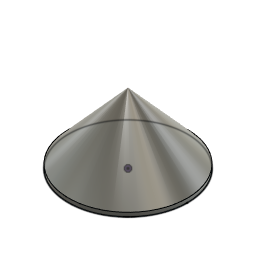
cylinderProjectFinal (Autodesk Fusion 360 design; units mm, degrees)
Autodesk Fusion 360 part; units mm, degrees
sketch "Sketch1" plane through (0, 0, 0) normal (0, 1, 0) x (1, 0, 0)
  circle A0 centre (0, 0) radius 45
  dimension "d1" = 90
  constraint coincident A0.centre origin
  measures "d1" diameter of A0
extrude "Extrude1" add sketch "Sketch1" along normal blind 100 makes body 1
sketch "Sketch2" plane through (0, 100, 0) normal (0, 1, 0) x (-1, 0, 0)
  circle A0 centre (0, 0) radius 45
  circle A1 centre (0, 0) radius 42.5
  dimension "d4" = 85
  constraint coincident A0.centre A1.centre
  measures "d4" diameter of A1
extrude "Extrude2" cut sketch "Sketch2" against normal blind 110 contours A1 bodies 1
sketch "Sketch3" plane through (0, 0, 0) normal (0, 0, 1) x (1, 0, 0)
extrude "Extrude3" add sketch "Sketch1" along normal blind 3 separate body makes body 2
sketch "Sketch4" plane through (0, 0, 0) normal (0, 0, 1) x (1, 0, 0)
  line L0 (0, 3) -> (0, 53)
  line L1 (0, 53) -> (45, 3)
  line L2 (45, 3) -> (0, 3)
  dimension "d9" = 50
  constraint vertical L0
  constraint perpendicular L0 L2
  measures "d9" distance of L0.start L0.end
revolve "Revolve1" add sketch "Sketch4" angle 360 about axis through (0, 3, 0) along (0, 1, 0) bodies 2
shell "Shell1" thickness 5 removed faces 1 at (4.1569, 0, 25.5535) on bodies 2
hidden bodies 1
